endplate (Autodesk Fusion 360 design; units mm, degrees)
Autodesk Fusion 360 part; units mm, degrees
sketch "Sketch1" plane through (0, 0, 0) normal (0, 1, 0) x (1, 0, 0)
  circle A0 centre (0, 0) radius 3
  circle A1 centre (0, 0) radius 5
  circle A2 centre (50, 0) radius 5
  circle A3 centre (50, 0) radius 3
  circle A4 centre (0, 50) radius 5
  circle A5 centre (0, 50) radius 3
  circle A6 centre (50, 50) radius 5
  circle A7 centre (50, 50) radius 3
  line L0 (0, 0) -> (0, 50) construction
  line L1 (0, 50) -> (50, 50) construction
  line L2 (50, 50) -> (50, 0) construction
  line L3 (50, 0) -> (0, 0) construction
  line L4 (50, 25) -> (25, 25) construction
  line L5 (25, 25) -> (25, 0) construction
  line L6 (50, 25) -> (60, 25) construction
  circle A8 centre (60, 25) radius 21.9258
  circle A9 centre (25, 60) radius 21.9258
  circle A10 centre (-10, 25) radius 21.9258
  circle A11 centre (25, -10) radius 21.9258
  circle A12 centre (25, 25) radius 13.0742 construction
  circle A13 centre (25, 25) radius 8.0742
  dimension "d1" = 6
  dimension "d2" = 10
  dimension "d5" = 50
  dimension "d6" = 50
  dimension "d7" = 10
  dimension "d9" = 360
  dimension "d10" = 5
  constraint coincident A0.centre A1.centre
  constraint concentric A0 A1
  constraint coincident A4.centre A5.centre
  constraint coincident A6.centre A7.centre
  constraint coincident A2.centre A3.centre
  constraint midpoint L2 L4.start
  constraint perpendicular L2 L4
  constraint midpoint L3 L5.end
  constraint perpendicular L3 L5
  constraint perpendicular L2 L6
  constraint coincident L6.end A8.centre
  constraint tangent A2 A8
  constraint coincident L4.end L5.start
  constraint tangent A10 A12
  constraint concentric A12 A13
  measures "d1" diameter of A0
  measures "d2" diameter of A1
  measures "d7" distance of L4.start L6.end
  measures "d10" distance of A12 A13
extrude "Extrude1" add sketch "Sketch1" along normal blind 10 contours A1 | A1 A2 A4 A6 A8 A9 A10 A11 | A4 | A2 | A6
